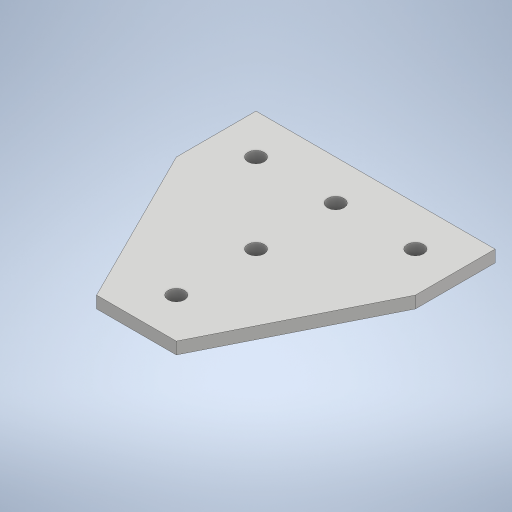
# Autodesk Inventor part: T
Saved by Autodesk Inventor 2024.2 (Build 282272000, 272)
## iProperties
Created: 2025-07-02
Part Number: T
Material: Genérico
Document SubType Name: Modeling
Designer: jd.castellanosq
Density: 1 g/cm^3
Appearance: Valor por defecto
Author: jd.castellanosq
Autodesk Inventor part; units mm, degrees
ref_plane "YZ Plane" through (0, 0, 0) normal (1, 0, 0) x (0, 1, 0)
ref_plane "XZ Plane" through (0, 0, 0) normal (0, 1, 0) x (-1, 0, 0)
ref_plane "XY Plane" through (0, 0, 0) normal (0, 0, 1) x (1, 0, 0)
sketch "Boceto1" plane through (0, 0, 0) normal (0, 0, 1) x (1, 0, 0)
  line L0 (-20, 0) -> (20, 0)
  line L1 (20, 0) -> (60, 80)
  line L2 (60, 80) -> (60, 120)
  line L3 (60, 120) -> (-60, 120)
  line L4 (-60, 120) -> (-60, 80)
  line L5 (-60, 80) -> (-20, 0)
  circle A0 centre (0, 100) radius 4.15
  circle A1 centre (0, 60) radius 4.15
  circle A2 centre (0, 20) radius 4.15
  circle A3 centre (40, 100) radius 4.15
  circle A4 centre (-40, 100) radius 4.15
  point P0 (0, 0)
  point P1 (0, 0)
  point P2 (0, 120)
  dimension "d0" = 120
  dimension "d1" = 120
  dimension "d2" = 40
  dimension "d3" = 40
  dimension "d4" = 20
  dimension "d5" = 8.3
  dimension "d6" = 40
  dimension "d7" = 40
  dimension "d8" = 40
  dimension "d9" = 40
  constraints: 12 end point, 5 centre point, 4 equal radius, 4 vertical alignment, 3 perpendicular, 2 coincident, 2 horizontal alignment, 2 midpoint, 1 horizontal, 1 parallel
  measures "d0" distance between parallel lines of L0 L3
  measures "d1" distance of L2.end L3.end
  measures "d2" distance of L1.end L2.end
  measures "d3" distance of L0.start L0.end
  measures "d4" distance from line of L3 A0.centre
  measures "d5" diameter of A0
  measures "d6" distance of A0.centre A4.centre
  measures "d7" distance of A3.centre A0.centre
  measures "d8" distance of A0.centre A1.centre
  measures "d9" distance of A2.centre A1.centre
extrude "Extrusión1" add sketch "Boceto1" along normal blind 6
equation "\"d8\" = d7"
equation "\"d9\" = d7"
